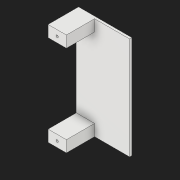
# Autodesk Inventor part: BP009
Saved by Autodesk Inventor 2017 SP1 (Build 210196100, 196)
## iProperties
Created: 2018-03-11
Part Number: BP009
Material: ABS Plastic
Document SubType Name: Modeling
Designer: Zach
Density: 1.06 g/cm^3
Appearance: CR White
Author: Zach
Autodesk Inventor part; units mm, degrees
ref_plane "YZ Plane" through (0, 0, 0) normal (1, 0, 0) x (0, 1, 0)
ref_plane "XZ Plane" through (0, 0, 0) normal (0, 1, 0) x (-1, 0, 0)
ref_plane "XY Plane" through (0, 0, 0) normal (0, 0, 1) x (1, 0, 0)
sketch "Sketch1" plane through (0, 0, 0) normal (0, 0, 1) x (1, 0, 0)
  line L0 (0, 0) -> (70, 0)
  line L1 (70, 0) -> (70, 134)
  line L2 (70, 134) -> (0, 134)
  line L3 (0, 134) -> (0, 0)
  dimension "d0" = 70
  dimension "d1" = 134
  constraints: 8 end point, 2 parallel, 1 horizontal, 1 perpendicular
  measures "d0" distance of L2.end L1.end
  measures "d1" distance of L1.end L0.end
extrude "Extrusion1" add sketch "Sketch1" along normal blind 3
sketch "Sketch2" plane through (0, 0, 3) normal (0, 0, 1) x (1, 0, 0)
  line L0 (70, 134) -> (0, 134) projected
  line L1 (0, 134) -> (24, 134)
  line L2 (24, 134) -> (24, 119)
  line L3 (24, 119) -> (0, 119)
  line L4 (0, 119) -> (0, 134)
  line L5 (0, 0) -> (24, 0)
  line L6 (24, 0) -> (24, 15)
  line L7 (24, 15) -> (0, 15)
  line L8 (0, 15) -> (0, 0)
  dimension "d4" = 24
  dimension "d5" = 15
  dimension "d6" = 24
  dimension "d7" = 15
  constraints: 16 end point, 4 parallel, 2 horizontal, 2 perpendicular
  measures "d4" distance of L2.end L3.end
  measures "d5" distance of L1.end L2.end
  measures "d6" distance of L7.end L6.end
  measures "d7" distance of L6.end L5.end
extrude "Extrusion2" add sketch "Sketch2" along normal blind 37
sketch "Sketch3" plane through (0, 0, 40) normal (0, 0, 1) x (1, 0, 0)
  line L0 (24, 134) -> (0, 134) construction
  line L1 (0, 134) -> (0, 119) construction
  line L2 (0, 119) -> (24, 119) construction
  line L3 (24, 119) -> (24, 134) construction
  line L4 (0, 0) -> (24, 0) construction
  line L5 (24, 0) -> (24, 15) construction
  line L6 (24, 15) -> (0, 15) construction
  line L7 (0, 15) -> (0, 0) construction
  circle A0 centre (12, 126.5) radius 1.5
  circle A1 centre (12, 7.5) radius 1.5
  point P0 (24, 126.5)
  point P1 (24, 7.5)
  point P2 (12, 15)
  point P3 (12, 119)
  dimension "d10" = 3
  dimension "d11" = 3
  constraints: 4 midpoint, 2 centre point, 2 horizontal alignment, 2 vertical alignment
  measures "d10" diameter of A0
  measures "d11" diameter of A1
extrude "Extrusion3" cut sketch "Sketch3" against normal through all
sketch "Sketch4" plane through (0, 0, 0) normal (0, 0, -1) x (-1, 0, 0)
  circle A0 centre (-12, 126.5) radius 1.5 projected
  circle A1 centre (-12, 7.5) radius 1.5 projected
  circle A2 centre (-12, 126.5) radius 4
  circle A3 centre (-12, 7.5) radius 4
  point P0 (0, 0)
  dimension "d14" = 8
  dimension "d15" = 8
  constraints: 2 centre point, 2 coincident
  measures "d14" diameter of A2
  measures "d15" diameter of A3
extrude "Extrusion4" cut sketch "Sketch4" against normal blind 35 contours A0 | A1 | A2 | A3
body "Solid1"
